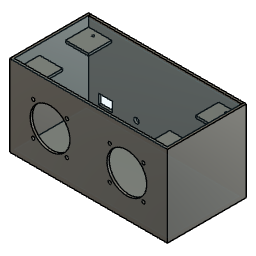
speaker (Autodesk Fusion 360 design; units mm, degrees)
Autodesk Fusion 360 part; units mm, degrees
sketch "Sketch4" plane through (0, 0, 0) normal (0, 0, 1) x (1, 0, 0)
  line L0 (200, 0) -> (0, 0)
  circle A0 centre (150, 50) radius 26
  line L1 (200, 100) -> (200, 0)
  circle A1 centre (49.695, 50) radius 26
  line L2 (0, 0) -> (0, 100)
  line L3 (0, 100) -> (200, 100)
  line L4 (49.695, 50) -> (49.695, 76)
  line L5 (49.695, 76) -> (75.695, 76)
  line L6 (75.695, 76) -> (75.695, 24)
  line L7 (75.695, 24) -> (23.695, 24)
  line L8 (23.695, 24) -> (23.695, 76)
  line L9 (49.695, 76) -> (23.695, 76)
  circle A2 centre (71.695, 72) radius 2.1
  line L10 (71.6806, 76) -> (71.695, 72)
  line L11 (71.695, 72) -> (75.695, 72)
  circle A3 centre (27.695, 72) radius 2.1
  circle A4 centre (27.695, 28) radius 2.1
  circle A5 centre (71.695, 28) radius 2.1
  circle A6 centre (171.695, 72) radius 2.1
  circle A7 centre (171.695, 28) radius 2.1
  circle A8 centre (127.695, 28) radius 2.1
  circle A9 centre (127.695, 72) radius 2.1
  point P0 (0, 100)
  dimension "d22" = 200
  dimension "d23" = 100
  dimension "d24" = 52
  dimension "d25" = 52
  dimension "d78" = 26
  dimension "d79" = 52
  dimension "d80" = 52
  dimension "d81" = 52
  dimension "d82" = 4.2
  dimension "d85" = 4
  dimension "d86" = 4
  dimension "d88" = 4.2
  dimension "d89" = 4.2
  dimension "d90" = 4.2
  dimension "d91" = 4.2
  dimension "d92" = 4.2
  dimension "d93" = 4.2
  dimension "d94" = 4.2
  constraint horizontal L3
  constraint vertical L1
  constraint horizontal L0
  constraint vertical L2
  constraint coincident P0 L2.end
  constraint coincident A1.centre L4.start
  constraint coincident A1 L4.end
  constraint perpendicular L3 L4
  constraint perpendicular L4 L5
  constraint perpendicular L5 L6
  constraint perpendicular L6 L7
  constraint perpendicular L7 L8
  constraint coincident L5 L10.start
  constraint coincident A2.centre L10.end
  constraint coincident L6 L11.end
  constraint perpendicular L6 L11
  measures "d22" distance of L1.start P0
  measures "d23" distance of P0 L0.end
  measures "d24" diameter of A1
  measures "d25" diameter of A0
  measures "d78" distance of L4.end L5.end
  measures "d79" distance of L5.end L6.end
  measures "d80" distance of L6.end L7.end
  measures "d81" distance of L7.end L8.end
  measures "d82" diameter of A2
  measures "d85" distance of A2.centre L11.end
  measures "d86" vertical distance of L10.start A2.centre
  measures "d88" diameter of A3
  measures "d89" diameter of A5
  measures "d90" diameter of A4
  measures "d91" diameter of A6
  measures "d92" diameter of A9
  measures "d93" diameter of A7
  measures "d94" diameter of A8
extrude "Extrude3" add sketch "Sketch4" against normal blind 3 contours L0 L1 L2 L3 | A1 L6 L7 | A1 L5 L6 A2 L10 L11 | A1 L8 L9 | A1 L7 L8 | L5 L6 A2 L10 L11 | A2 L10 L11 | A2 L10 L11 | A3 | A4 | A5 | A6 | A7 | A8 | A9 makes body 1
sketch "Sketch6" plane through (0, 0, 0) normal (0, 1, 0) x (1, 0, 0)
  line L0 (0, 0) -> (0, 3)
  line L1 (0, 3) -> (200, 3)
  line L2 (200, 3) -> (200, 100)
  line L3 (200, 100) -> (0, 100)
  line L4 (0, 100) -> (0, 3)
  dimension "d30" = 3
  dimension "d31" = 200
  dimension "d32" = 97
  constraint coincident L0.start origin
  constraint vertical L0
  constraint horizontal L1
  constraint vertical L2
  constraint horizontal L3
  constraint vertical L4
  measures "d30" distance of L0.start L0.end
  measures "d31" distance of L0.end L1.end
  measures "d32" distance of L0.end L3.end
extrude "Extrude4" add sketch "Sketch6" along normal blind 3 separate body makes body 2
copy_body "CopyPasteBodies1" bodies 2 makes body 3
move_body "Move1" bodies 3 to x (1, 0, 0) y (0, 1, 0) z (0, 0, 1) at (0, 97, 0)
sketch "Sketch7" plane through (0, 0, 0) normal (1, 0, 0) x (0, 0, -1)
  line L0 (0, 0) -> (3, 0)
  line L1 (3, 0) -> (3, 3)
  line L2 (3, 3) -> (97, 3)
  line L3 (97, 3) -> (97, 97)
  line L4 (97, 97) -> (3, 97)
  line L5 (3, 97) -> (3, 3)
  dimension "d35" = 3
  dimension "d36" = 3
  dimension "d37" = 94
  dimension "d38" = 94
  constraint coincident L0.start origin
  constraint horizontal L0
  constraint perpendicular L0 L1
  constraint horizontal L2
  constraint vertical L3
  constraint horizontal L4
  constraint vertical L5
  measures "d35" distance of L0.start L0.end
  measures "d36" distance of L0.end L1.end
  measures "d37" distance of L1.end L2.end
  measures "d38" distance of L1.end L4.end
extrude "Extrude5" add sketch "Sketch7" along normal blind 3 separate body makes body 4
copy_body "CopyPasteBodies2" bodies 4 makes body 5
move_body "Move2" bodies 5 to x (1, 0, 0) y (0, 1, 0) z (0, 0, 1) at (197, 0, 0)
sketch "Sketch8" plane through (0, 0, 0) normal (0, 0, 1) x (1, 0, 0)
  line L0 (0, 0) -> (200, 0)
  line L1 (200, 0) -> (200, 100)
  line L2 (200, 100) -> (0, 100)
  line L3 (0, 100) -> (0, 0)
  dimension "d41" = 200
  dimension "d42" = 100
  constraint horizontal L0
  constraint vertical L1
  constraint horizontal L2
  constraint vertical L3
  constraint coincident L0.start L3.end
  measures "d41" distance of L0.start L0.end
  measures "d42" distance of L0.start L2.end
extrude "Extrude6" add sketch "Sketch8" along normal blind 3 separate body makes body 6
move_body "Move3" bodies 6 to x (1, 0, 0) y (0, 1, 0) z (0, 0, 1) at (0, 0, -165)
move_body "Move4" bodies 6 to x (1, 0, 0) y (0, 1, 0) z (0, 0, 1) at (0, 0, 65)
move_body "Move5" bodies 3 to x (1, 0, 0) y (0, 1, 0) z (0, 0, 1) at (0, 3, 0)
move_body "Move6" bodies 3 to x (1, 0, 0) y (0, 1, 0) z (0, 0, 1) at (0, 0, 3)
move_body "Move7" bodies 2 to x (1, 0, 0) y (0, 1, 0) z (0, 0, 1) at (0, -3, 0)
move_body "Move8" bodies 2 to x (1, 0, 0) y (0, 1, 0) z (0, 0, 1) at (0, 0, 3)
move_body "Move9" bodies 5 to x (1, 0, 0) y (0, 1, 0) z (0, 0, 1) at (3, 0, 0)
move_body "Move10" bodies 5 to x (1, 0, 0) y (0, 1, 0) z (0, 0, 1) at (0, -6, 0)
move_body "Move11" bodies 5 to x (1, 0, 0) y (0, 1, 0) z (0, 0, 1) at (0, 0, 3)
extrude "Extrude7" add 1 faces at (201, 91, -62.6667) along direction (0, 1, 0) blind 12 on bodies 5 bodies 5
move_body "Move12" bodies 4 to x (1, 0, 0) y (0, 1, 0) z (0, 0, 1) at (-3, 0, 0)
extrude "Extrude8" add 1 faces at (-2, 97, -65.6667) along direction (0, 1, 0) blind 6 on bodies 4 bodies 4
extrude "Extrude9" add 1 faces at (-2, 3, -34.3333) along direction (0, -1, 0) blind 6 on bodies 4 bodies 4
move_body "Move13" bodies 4 to x (1, 0, 0) y (0, 1, 0) z (0, 0, 1) at (0, 0, 3)
move_body "Move14" bodies 6 to x (1, 0, 0) y (0, 1, 0) z (0, 0, 1) at (0, 0, 6)
copy_body "CopyPasteBodies3" bodies 3 makes body 7
move_body "Move15" bodies 7 to x (1, 0, 0) y (0, 1, 0) z (0, 0, 1) at (0, -3, 0)
extrude "Extrude10" cut 1 faces at (66.6667, 98, 0) along direction (0, 0, -1) blind 3 on bodies 7 bodies 7
extrude "Extrude11" cut 1 faces at (133.3333, 98, -97) along direction (0, 0, 1) blind 3 on bodies 7 bodies 7
copy_body "CopyPasteBodies4" bodies 7 makes body 8
move_body "Move16" bodies 8 to x (1, 0, 0) y (0, 1, 0) z (0, 0, 1) at (0, -97, 0)
extrude "Extrude12" add 1 faces at (66.6667, 3, -63.6667) along direction (0, 1, 0) blind 2 on bodies 8 bodies 8
extrude "Extrude13" add 1 faces at (66.6667, 97, -63.6667) along direction (0, -1, 0) blind 2 on bodies 7 bodies 7
sketch "Sketch10" plane through (0, 0, -94) normal (0, 0, -1) x (-1, 0, 0)
  line L0 (-200, 0) -> (0, 0)
  line L1 (0, 0) -> (0, 5)
  line L2 (0, 5) -> (-200, 5)
  line L3 (-200, 5) -> (-200, 0)
  line L4 (-200, 0) -> (-195, 0)
  line L5 (-195, 0) -> (-195, 2.5)
  circle A0 centre (-195, 2.5) radius 1.5
  dimension "d61" = 5
  dimension "d62" = 2.5
  dimension "d63" = 3
  constraint coincident L0.start L3.end
  constraint perpendicular L3 L4
  constraint perpendicular L4 L5
  constraint coincident L5.end A0.centre
  measures "d61" distance of L0.start L4.end
  measures "d62" distance of L4.end L5.end
  measures "d63" diameter of A0
copy_body "CopyPasteBodies5" bodies 5 makes body 9
move_body "Move17" bodies 9 to x (1, 0, 0) y (0, 1, 0) z (0, 0, 1) at (-3, 0, 0)
extrude "Extrude14" cut 1 faces at (198, -3, -31.3333) along direction (0, 1, 0) blind 8 on bodies 9 bodies 9
extrude "Extrude15" cut 1 faces at (198, 37.6667, -94) along direction (0, 0, 1) blind 3 on bodies 9 bodies 9
extrude "Extrude16" cut 1 faces at (198, 70.3333, 0) along direction (0, 0, -1) blind 3 on bodies 9 bodies 9
extrude "Extrude17" cut 1 faces at (198, 103, -61.6667) along direction (0, -1, 0) blind 8 on bodies 9 bodies 9
extrude "Extrude18" add 1 faces at (197, 35, -32.3333) along direction (-1, 0, 0) blind 2 on bodies 9 bodies 9
copy_body "CopyPasteBodies6" bodies 9 makes body 10
move_body "Move18" bodies 10 to x (1, 0, 0) y (0, 1, 0) z (0, 0, 1) at (-195, 0, 0)
sketch "Sketch11" plane through (0, 103, 0) normal (0, 1, 0) x (-1, 0, 0)
  line L0 (0, -97) -> (0, 0)
  line L1 (0, 0) -> (-200, 0)
  line L2 (-200, 0) -> (-200, -97)
  line L3 (-200, -97) -> (0, -97)
move_body "Move22" bodies 6 to x (1, 0, 0) y (0, 1, 0) z (0, 0, 1) at (0, 0, -3)
extrude "Extrude20" add 1 faces at (-1, 32.3333, -94) along direction (0, 0, -1) blind 3 on bodies 4 bodies 4
extrude "Extrude21" add 1 faces at (201, 32.3333, -94) along direction (0, 0, -1) blind 3 on bodies 5 bodies 5
extrude "Extrude22" cut sketch "Sketch4" against normal blind 5 contours A2 L10 L11 | A2 L10 L11 | A3 | A4 | A5 | A6 | A7 | A8 | A9 bodies 1
extrude "Extrude23" cut 1 faces at (66.6667, -2, 0) along direction (0, 0, -1) blind 3 on bodies 2 bodies 2
extrude "Extrude24" add 1 faces at (133.3333, 0, -1) along direction (0, -1, 0) blind 3 on bodies 1 bodies 1 2 4 5
extrude "Extrude25" add 1 faces at (66.6667, 100, -1) along direction (0, 1, 0) blind 3 on bodies 1 bodies 1
sketch "Sketch12" plane through (0, 0, 0) normal (1, 0, 0) x (0, 0, -1)
  line L0 (3, 103) -> (3, 0)
  line L1 (3, 0) -> (97, 0)
  line L2 (97, 0) -> (97, 103)
  line L3 (97, 103) -> (3, 103)
  line L4 (97, 103) -> (97, 90)
  line L5 (97, 90) -> (0, 90)
  line L6 (3, 90) -> (3, 87)
  line L7 (3, 87) -> (6, 87)
  line L8 (6, 87) -> (6, 90)
  line L9 (97, 90) -> (97, 87)
  dimension "d107" = 13
  dimension "d108" = 97
  dimension "d109" = 3
  dimension "d110" = 3
  dimension "d111" = 3
  constraint coincident L2.end L3.start
  constraint perpendicular L3 L4
  constraint perpendicular L0 L5
  constraint coincident L5 L6.start
  constraint coincident L0 L6.start
  constraint perpendicular L5 L6
  constraint perpendicular L6 L7
  constraint coincident L5 L8.end
  constraint perpendicular L5 L8
  constraint perpendicular L5 L9
  measures "d107" distance of L2.end L4.end
  measures "d108" distance of L4.end L5.end
  measures "d109" distance of L6.start L6.end
  measures "d110" distance of L6.end L7.end
  measures "d111" distance of L4.end L9.end
sketch "Sketch13" plane through (0, 51.5, -50) normal (1, 0, 0) x (0, 0, -1)
extrude "Extrude26" add sketch "Sketch12" along normal blind 30 separate body contours L0 L5 L6 L7 L8 makes body 11
extrude "Extrude27" add 1 faces at (20, 88, -6) along direction (0, 0, -1) blind 30 on bodies 11 bodies 11
sketch "Sketch14" plane through (0, 90, 0) normal (0, 1, 0) x (-1, 0, 0)
  line L0 (0, -36) -> (0, -3)
  line L1 (0, -3) -> (-30, -3)
  line L2 (-30, -3) -> (-30, -36)
  line L3 (-30, -36) -> (0, -36)
  line L4 (0, -3) -> (-13, -3)
  line L5 (-13, -3) -> (-13, -13)
  circle A0 centre (-13, -13) radius 1.6
  dimension "d116" = 13
  dimension "d117" = 10
  dimension "d118" = 3.2
  constraint coincident L0.end L1.start
  constraint perpendicular L0 L4
  constraint perpendicular L4 L5
  constraint coincident L5.end A0.centre
  measures "d116" distance of L0.end L4.end
  measures "d117" distance of L4.end L5.end
  measures "d118" diameter of A0
extrude "Extrude28" cut sketch "Sketch14" against normal blind 7.5 contours A0 bodies 11
sketch "Sketch15" plane through (0, 0, 0) normal (0, 1, 0) x (-1, 0, 0)
  line L0 (0, -3) -> (-200, -3)
  line L1 (-200, -3) -> (-200, -97)
  line L2 (-200, -97) -> (0, -97)
  line L3 (0, -97) -> (0, -3)
copy_body "CopyPasteBodies9" bodies 11 makes body 12
move_body "Move29" bodies 12 to x (1, 0, 0) y (0, 1, 0) z (0, 0, 1) at (170, 0, 0)
move_body "Move30" bodies 12 to x (-1, 0, 0) y (0, -1, 0) z (0, 0, 1) at (340, 174, 0)
move_body "Move31" bodies 12 to x (1, 0, 0) y (0, 1, 0) z (0, 0, 1) at (30, 0, 0)
copy_body "CopyPasteBodies10" bodies 12 11 makes body 13 makes body 14
move_body "Move32" bodies 13 14 to x (1, 0, 0) y (0, -1, 0) z (0, 0, -1) at (0, 168, -100)
move_body "Move33" bodies 14 to x (1, 0, 0) y (0, 1, 0) z (0, 0, 1) at (0, 9, 0)
move_body "Move34" bodies 13 to x (1, 0, 0) y (0, 1, 0) z (0, 0, 1) at (0, 3, 0)
move_body "Move35" bodies 13 12 to x (1, 0, 0) y (0, 1, 0) z (0, 0, 1) at (0, 3, 0)
extrude "Extrude29" add 1 faces at (133.3333, 100, -96) along direction (0, 1, 0) blind 3 on bodies 6 bodies 6
extrude "Extrude30" cut 2 faces at (180, 89, -97) (20, 88, -97) along direction (0, 0, 1) blind 3 on bodies 13 14 bodies 13 14
extrude "Extrude31" add 1 faces at (66.6667, -2, -97) along direction (0, 0, -1) blind 6 on bodies 1 bodies 1
move_body "Move36" bodies 13 14 to x (1, 0, 0) y (0, 1, 0) z (0, 0, 1) at (0, 0, -6)
move_body "Move37" bodies 6 to x (1, 0, 0) y (0, 1, 0) z (0, 0, 1) at (0, 0, -6)
sketch "Sketch16" plane through (0, 0, -103) normal (0, 0, -1) x (-1, 0, 0)
  line L0 (0, 0) -> (0, 103)
  line L1 (0, 103) -> (-200, 103)
  line L2 (-200, 103) -> (-200, 0)
  line L3 (-200, 0) -> (0, 0)
  line L4 (-31.124, 21.5395) -> (-13.124, 21.5395)
  line L5 (-13.124, 21.5395) -> (-13.124, 8.5395)
  line L6 (-13.124, 8.5395) -> (-31.124, 8.5395)
  line L7 (-31.124, 8.5395) -> (-31.124, 21.5395)
  circle A0 centre (-62.5707, 15.2017) radius 3.5
  dimension "d127" = 18
  dimension "d128" = 13
  dimension "d129" = 7
  constraint horizontal L4
  constraint vertical L5
  constraint horizontal L6
  constraint vertical L7
  measures "d127" distance of L4.start L4.end
  measures "d128" distance of L4.start L6.end
  measures "d129" diameter of A0
extrude "Extrude32" cut sketch "Sketch16" against normal blind 10 contours L4 L5 L6 L7 | A0 bodies 6
hidden bodies 3 7 8 9 10
